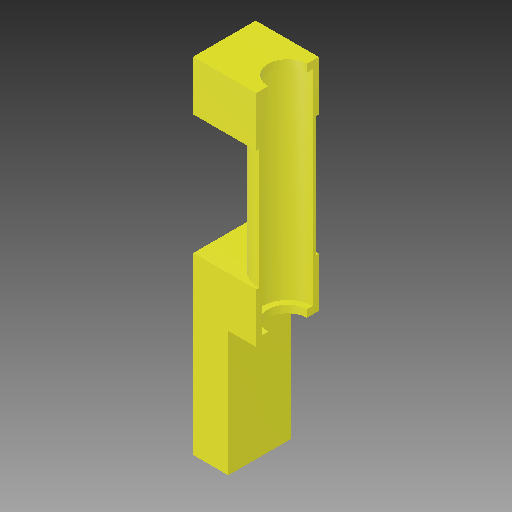
# Autodesk Inventor part: 蓋子加平面2
Saved by Autodesk Inventor 2017 (Build 210142000, 142)
## iProperties
Created: 2019-12-03
Part Number: 蓋子加平面2
Material: 一般
Document SubType Name: Modeling
Designer: 吳昇峻
Density: 1 g/cm^3
Appearance: White Ash - Java
Mass: 39.2248 g
Surface Area: 137.846 cm^2
Volume: 39.2248 cm^3
Author: 吳昇峻
Autodesk Inventor part; units mm, degrees
ref_plane "YZ Plane" through (0, 0, 0) normal (1, 0, 0) x (0, 1, 0)
ref_plane "XZ Plane" through (0, 0, 0) normal (0, 1, 0) x (-1, 0, 0)
ref_plane "XY Plane" through (0, 0, 0) normal (0, 0, 1) x (1, 0, 0)
sketch "草圖1" plane through (0, 0, 0) normal (0, 1, 0) x (-1, 0, 0)
  arc A0 (0, -10) -> (0, 10) centre (0, 0) ccw
  arc A1 (0, -11.5) -> (0, 11.5) centre (0, 0) ccw
  line L0 (0, 11.5) -> (0, 10)
  line L1 (0, -10) -> (0, -11.5)
  dimension "d0" = 20
  dimension "d1" = 23
  constraints: 4 end point, 4 point on circle, 2 centre point, 2 coincident, 2 point on line, 1 vertical
  measures "d0" diameter of A0
  measures "d1" diameter of A1
extrude "擠出1" add sketch "草圖1" along normal blind 40
sketch "草圖2" plane through (0, 40, 0) normal (0, 1, 0) x (1, 0, 0)
  line L0 (0, -11.5) -> (0, -10) projected
  arc A0 (0, 11.5) -> (0, -11.5) centre (0, 0) ccw projected
  line L1 (0, 10) -> (0, 11.5) projected
  line L2 (0, -10) -> (0, 10)
  constraints: 2 end point, 1 vertical
extrude "擠出2" add sketch "草圖2" along normal blind 3
sketch "草圖3" plane through (0, 43, 0) normal (0, 1, 0) x (1, 0, 0)
  arc A0 (0, 7.75) -> (0, -7.75) centre (0, 0) ccw
  line L0 (0, -10) -> (0, 10) projected
  line L1 (0, -7.75) -> (0, 7.75)
  dimension "d7" = 15.5
  constraints: 2 end point, 2 point on circle, 2 point on line, 1 centre point, 1 coincident
  measures "d7" diameter of A0
extrude "擠出3" cut sketch "草圖3" against normal up to next
sketch "草圖5" plane through (0, 0, 0) normal (0, -1, 0) x (1, 0, 0)
  arc A0 (0, 10) -> (0, -10) centre (0, 0) ccw projected
  line L0 (0, 10) -> (0, 11.5) projected
  arc A1 (0, 11.5) -> (0, -11.5) centre (0, 0) ccw projected
  line L1 (0, -11.5) -> (0, -10) projected
  line L2 (0, 11.5) -> (0, -11.5)
  constraints: 2 end point, 1 vertical
extrude "擠出4" add sketch "草圖5" along normal blind 3
sketch "草圖7" plane through (0, -3, 0) normal (0, -1, 0) x (1, 0, 0)
  arc A0 (0, 7.75) -> (0, -7.75) centre (0, 0) ccw
  line L0 (0, -11.5) -> (0, 11.5) projected
  line L1 (0, -7.75) -> (0, 7.75)
  dimension "d13" = 15.5
  constraints: 2 end point, 2 point on circle, 2 point on line, 1 centre point, 1 coincident
  measures "d13" diameter of A0
extrude "擠出5" cut sketch "草圖7" against normal up to next
sketch "草圖9" plane through (0, 0, 0) normal (0, 0, 1) x (1, 0, 0)
  line L0 (0, 43) -> (0, -3) construction
  line L1 (0, -3) -> (-11.2, -3) construction
  line L2 (-11.5, -3) -> (0, -3) construction
  line L3 (-11.2, -3) -> (-11.2, -103) construction
  line L4 (-11.2, -3) -> (-11.2, 17) construction
  line L5 (-11.2, 17) -> (-16.2, 17)
  line L6 (-16.2, 17) -> (-16.2, -123)
  line L7 (-16.2, -123) -> (-11.2, -123)
  line L8 (-11.2, -123) -> (-11.2, 17)
  point P0 (0, 0)
  dimension "d18" = 11.2
  dimension "d19" = 100
  dimension "d20" = 20
  dimension "d21" = 5
  dimension "d22" = 140
  dimension "d23" = 5
  constraints: 14 end point, 4 perpendicular, 1 horizontal, 1 point on line
  measures "d18" distance of L0.end L1.end
  measures "d19" distance of L1.end L3.end
  measures "d20" distance of L1.end L4.end
  measures "d21" distance of L4.end L5.end
  measures "d22" distance of L5.end L6.end
  measures "d23" distance of L6.end L7.end
extrude "擠出6" add sketch "草圖9" along normal mid plane 25
sketch "草圖11" plane through (0, -3, 0) normal (0, -1, 0) x (1, 0, 0)
  line L0 (-16.2, -12.5) -> (-11.2, -12.5) projected
  line L1 (-16.2, -12.5) -> (0, -12.5)
  line L2 (-11.2, -12.5) -> (-16.2, -12.5) projected
  line L3 (-16.2, -12.5) -> (-16.2, 12.5) projected
  line L4 (-16.2, 12.5) -> (-11.2, 12.5) projected
  line L5 (-11.2, 12.5) -> (0, 12.5)
  line L6 (0, 12.5) -> (0, 11.5)
  arc A0 (-11.2, -2.6096) -> (0, -11.5) centre (0, 0) ccw projected
  arc A1 (0, 11.5) -> (-11.2, 2.6096) centre (0, 0) ccw projected
  line L7 (-11.2, -12.5) -> (-11.2, 12.5) projected
  line L8 (0, -12.5) -> (0, -11.5)
  constraints: 8 end point, 2 horizontal, 1 perpendicular, 1 vertical
extrude "擠出7" add sketch "草圖11" against normal blind 20 contours L7 A0 L8 L1 | L5 L6 A1 L7
sketch "草圖12" plane through (-11.2, -123, 12.5) normal (1, 0, 0) x (0, 0, -1)
  line L0 (20.25, 120) -> (4.75, 120) construction
  line L1 (25, 120) -> (0, 120) projected
  line L2 (0, 0) -> (0, 120) projected
  line L3 (25, 0) -> (0, 0) projected
  line L4 (25, 120) -> (25, 0) projected
  line L5 (0, 120) -> (0, 70) construction
  line L6 (0, 70) -> (25, 70)
  point P0 (12.5, 123)
  dimension "d36" = 50
  constraints: 4 end point, 2 point on line, 1 perpendicular
  measures "d36" distance of L1.end L5.end
extrude "擠出9" cut sketch "草圖12" against normal up to next contours L4 L3 L2 L6
sketch "草圖16" plane through (0, 43, 0) normal (0, 1, 0) x (1, 0, 0)
  arc A0 (0, 10) -> (0, -10) centre (0, 0) ccw projected
  arc A1 (0, 11.5) -> (0, -11.5) centre (0, 0) ccw projected
  line L0 (0, -11.5) -> (0, -7.75) projected
  line L1 (0, 7.75) -> (0, 11.5) projected
extrude "擠出11" add sketch "草圖16" along normal blind 39
sketch "草圖17" plane through (0, 82, 0) normal (0, 1, 0) x (1, 0, 0)
  line L0 (0, -10) -> (0, -7.75) projected
  arc A0 (0, 7.75) -> (0, -7.75) centre (0, 0) ccw projected
  line L1 (0, 7.75) -> (0, 10) projected
  arc A1 (0, 11.5) -> (0, -11.5) centre (0, 0) ccw projected
  line L2 (0, -11.5) -> (0, -10) projected
  line L3 (0, 10) -> (0, 11.5) projected
extrude "擠出12" add sketch "草圖17" along normal blind 3
sketch "草圖18" plane through (0, 85, 0) normal (0, 1, 0) x (1, 0, 0)
  arc A0 (0, 11.5) -> (0, -11.5) centre (0, 0) ccw projected
  line L0 (0, 11.5) -> (0, 12.5) projected
  line L1 (-16.2, 12.5) -> (0, 12.5) projected
  line L2 (-16.2, 12.5) -> (-16.2, -12.5) projected
  line L3 (-16.2, -12.5) -> (0, -12.5) projected
  line L4 (0, -12.5) -> (0, -11.5) projected
extrude "擠出13" add sketch "草圖18" against normal blind 20
sketch "草圖19" plane through (0, 43, 0) normal (0, 1, 0) x (1, 0, 0)
  arc A0 (0, 10) -> (0, -10) centre (0, 0) ccw projected
  line L0 (0, -10) -> (0, -7.75) projected
  arc A1 (0, 7.75) -> (0, -7.75) centre (0, 0) ccw projected
  line L1 (0, 7.75) -> (0, 10) projected
extrude "擠出14" cut sketch "草圖19" against normal blind 3
sketch "Sketch20" plane through (0, 0, 0) normal (0, 0, 1) x (1, 0, 0)
  line L0 (-11.2, -3) -> (0, -3) projected
  line L1 (0, 85) -> (-16.2, 85) projected
  point P0 (0, 0)
  dimension "d52" = 88
  measures "d52" distance between parallel lines of L0 L1
sketch "Sketch21" plane through (-16.2, 85, -12.5) normal (-1, 0, 0) x (0, 0, 1)
  line L0 (25, 0) -> (20.25, 0) projected
  line L1 (0, -20) -> (1, -20) projected
  line L2 (25, 0) -> (0, 0)
  line L3 (0, 0) -> (0, -20)
  line L4 (0, -20) -> (25, -20)
  line L5 (25, -20) -> (25, 0)
  line L6 (25, -68) -> (25, -138) projected
  line L7 (0, -138) -> (25, -138) projected
  line L8 (25, -68) -> (0, -68)
  line L9 (0, -68) -> (0, -138)
  line L10 (0, -138) -> (25, -138)
  line L11 (25, -138) -> (25, -68)
  point P0 (12.5, -85)
  constraints: 16 end point, 4 parallel, 2 horizontal, 2 perpendicular
extrude "Extrusion15" add sketch "Sketch21" along normal blind 9
